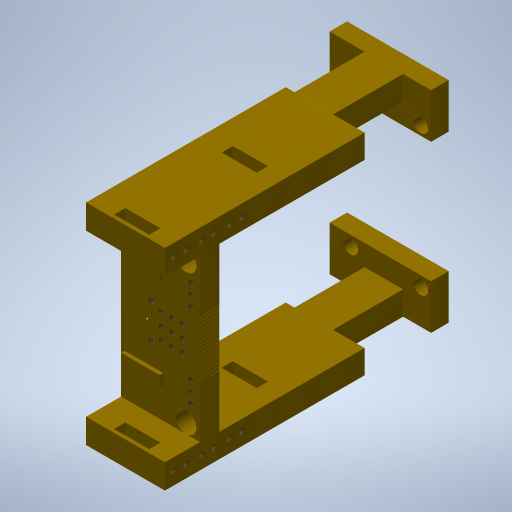
# Autodesk Inventor part: sample_holder_test
Saved by Autodesk Inventor 2024 (Build 280153000, 153)
## iProperties
Created: 2017-12-08
Part Number: sample_holder_test
Material: Generic
Document SubType Name: Modeling
Designer: awallucks
Density: 1 g/cm^3
Appearance: Default
Author: awallucks
Autodesk Inventor part; units mm, degrees
ref_plane "YZ Plane" through (0, 0, 0) normal (1, 0, 0) x (0, 1, 0)
ref_plane "XZ Plane" through (0, 0, 0) normal (0, 1, 0) x (-1, 0, 0)
ref_plane "XY Plane" through (0, 0, 0) normal (0, 0, 1) x (1, 0, 0)
sketch "Sketch1" plane through (0, 0, 0) normal (0, 1, 0) x (-1, 0, 0)
  line L0 (15, 30) -> (-15, 30)
  line L1 (-15, 30) -> (-15, -30)
  line L2 (-15, -30) -> (15, -30)
  line L3 (15, -30) -> (15, 30)
  point P0 (0, 0)
  dimension "d0" = 15
  dimension "d1" = 30
  dimension "d2" = 60
  dimension "d3" = 30
  constraints: 8 end point, 2 parallel, 1 horizontal, 1 perpendicular
  measures "d0" distance from line of L3 point (0, 0)
  measures "d1" distance between parallel lines of L1 L3
  measures "d2" distance between parallel lines of L2 L0
  measures "d3" distance from line of L0 point (0, 0)
extrude "Extrusion1" add sketch "Sketch1" along normal blind 72
sketch "Sketch2" plane through (0, 72, 0) normal (0, 1, 0) x (1, 0, 0)
  line L0 (15, 17.25) -> (15, -17.25)
  line L1 (-15, 30) -> (-15, -30) projected
  line L2 (15, 17.25) -> (-15, 17.25)
  line L3 (-15, 17.25) -> (-15, -17.25)
  line L4 (-15, -17.25) -> (15, -17.25)
  line L5 (15, -17.25) -> (15, 17.25)
  point P0 (0, 0)
  constraints: 10 end point, 2 parallel, 1 horizontal, 1 perpendicular, 1 point on line
extrude "Extrusion2" cut sketch "Sketch2" against normal blind 66.5
sketch "Sketch3" plane through (0, 72, 0) normal (0, 1, 0) x (1, 0, 0)
  circle A0 centre (11, -20) radius 2.15
  point P0 (0, 0)
  dimension "d15" = 20
  dimension "d16" = 11
  dimension "d17" = 4.3
  constraints: 1 centre point
  measures "d15" vertical distance of A0.centre point (0, 0)
  measures "d16" horizontal distance of A0.centre point (0, 0)
  measures "d17" diameter of A0
sketch "Sketch4" plane through (0, 72, 0) normal (0, 1, 0) x (1, 0, 0)
  point P0 (0, 0)
extrude "Extrusion3" cut sketch "Sketch3" against normal blind 50
pattern_linear "Rectangular Pattern1" count 2 spacing 20 along (-1, 0, 0) count 2 spacing 40 along (0, 0, -1) of "Extrusion3"
sketch "Sketch7" plane through (0, 5.5, 0) normal (0, 1, 0) x (1, 0, 0)
  line L0 (15, 17.25) -> (15, -17.25) projected
  line L1 (-15, -30) -> (15, -30) projected
  point P0 (0, 0)
  point P1 (1.2, -5)
  point P2 (1.2, 5)
  dimension "d47" = 13.8
  dimension "d51" = 10
  dimension "d85" = 5
  constraints: 1 vertical, 1 other
  measures "d47" distance from line of L0 point (1.2, -5)
  measures "d51" distance of point (1.2, -5) point (1.2, 5)
  measures "d85" vertical distance of point (0, 0) point (1.2, -5)
hole "Hole2" at (1.2, 5.5, 5) at (1.2, 5.5, -5) direction (0, -1, 0) diameter 1.567 depth 6.3 thread size "M2x0.4" class "6H" standard "ISO Metric profile"
sketch "Sketch10" plane through (15, 0, 30) normal (1, 0, 0) x (0, 0, -1)
  line L0 (0, 72) -> (12.75, 72)
  line L1 (12.75, 72) -> (12.75, 5.5)
  line L2 (12.75, 5.5) -> (0, 5.5)
  line L3 (0, 5.5) -> (0, 72)
  line L4 (60, 0) -> (60, 72) projected
  line L5 (47.25, 72) -> (60, 72)
  line L6 (60, 72) -> (60, 5.5)
  line L7 (60, 5.5) -> (47.25, 5.5)
  line L8 (47.25, 5.5) -> (47.25, 72)
  point P0 (30, 0)
  constraints: 16 end point, 4 parallel, 2 horizontal, 2 perpendicular, 2 point on line
extrude "Extrusion6" cut sketch "Sketch10" against normal blind 1
sketch "Sketch12" plane through (0, 0, 0) normal (0, -1, 0) x (1, 0, 0)
  line L0 (15, 6) -> (15, -6) projected
  line L1 (15, 30) -> (15, -30) projected
  point P0 (0, 0)
  point P1 (15, 0)
  point P2 (15, -1)
  point P3 (15, -2)
  point P4 (15, -3)
  point P5 (15, -4)
  point P6 (15, -5)
  point P7 (15, 0)
  point P8 (15, 1)
  point P9 (15, 2)
  point P10 (15, 3)
  point P11 (15, 4)
  point P12 (15, 5)
  point P13 (15, 0)
  point P14 (15, -7)
  point P15 (15, -8)
  point P16 (15, 7)
  point P17 (15, 8)
  dimension "d292" = 1
  dimension "d293" = 1
  dimension "d294" = 1
  dimension "d295" = 1
  dimension "d296" = 1
  constraints: 3 coincident, 15 other
  measures "d292" distance of point (15, 5) point (15, 6)
  measures "d293" distance of point (15, 7) point (15, 6)
  measures "d294" distance of point (15, -7) point (15, -6)
  measures "d295" distance of point (15, -8) point (15, -7)
  measures "d296" distance of point (15, 8) point (15, 7)
hole "Hole4" at (15, 0, 0) at (15, 0, -1) at (15, 0, -2) at (15, 0, -3) at (15, 0, 1) at (15, 0, 2) at (15, 0, 3) at (15, 0, -4) at (15, 0, -5) at (15, 0, 5) at (15, 0, 4) at (15, 0, 6) at (15, 0, -6) at (15, 0, -7) at (15, 0, -8) at (15, 0, 7) at (15, 0, 8) direction (0, 1, 0) diameter 0.2 end through all
sketch "Sketch14" plane through (15, 0, -30) normal (0, 0, -1) x (-1, 0, 0)
  line L0 (1, 67) -> (9, 67)
  line L1 (9, 67) -> (9, 47)
  line L2 (9, 47) -> (1, 47)
  line L3 (1, 47) -> (1, 67)
  line L4 (1, 67) -> (9, 47) construction
  line L5 (9, 67) -> (1, 47) construction
  line L6 (1, 72) -> (30, 72) projected
  line L7 (28, 47) -> (20, 47)
  line L8 (20, 47) -> (20, 67)
  line L9 (20, 67) -> (28, 67)
  line L10 (28, 67) -> (28, 47)
  line L11 (28, 47) -> (20, 67) construction
  line L12 (20, 47) -> (28, 67) construction
  line L13 (1, 72) -> (1, 5.5) projected
  line L14 (30, 0) -> (30, 72) projected
  point P0 (15, 0)
  point P1 (5, 57)
  point P2 (5, 67)
  point P3 (24, 57)
  point P4 (24, 47)
  dimension "d113" = 5
  dimension "d114" = 20
  dimension "d115" = 0
  dimension "d116" = 5
  dimension "d117" = 20
  dimension "d118" = 8
  dimension "d119" = 8
  dimension "d120" = 2
  constraints: 24 end point, 6 midpoint, 4 parallel, 2 horizontal, 2 perpendicular
  measures "d113" distance from line of point (5, 67) L6
  measures "d114" distance between parallel lines of L2 L0
  measures "d115" distance between parallel lines of L13 L3
  measures "d116" distance between parallel lines of L6 L9
  measures "d117" distance from line of point (24, 47) L9
  measures "d118" distance between parallel lines of L3 L1
  measures "d119" distance between parallel lines of L10 L8
  measures "d120" distance between parallel lines of L14 L10
extrude "Extrusion7" cut sketch "Sketch14" against normal blind 60
sketch "Sketch15" plane through (6, 47, 17.25) normal (0, 1, 0) x (1, 0, 0)
  line L0 (8, 0) -> (8, -12.75) projected
  line L1 (0, 0) -> (8, 0)
  line L2 (8, 0) -> (8, -6)
  line L3 (8, -6) -> (0, -6)
  line L4 (0, -6) -> (0, 0)
  line L5 (0, 0) -> (8, -6) construction
  line L6 (8, 0) -> (0, -6) construction
  line L7 (0, 0) -> (0, -12.75) projected
  line L8 (0, 0) -> (8, 0) projected
  line L9 (8, 40.5) -> (0, 40.5)
  line L10 (0, 40.5) -> (0, 34.5)
  line L11 (0, 34.5) -> (8, 34.5)
  line L12 (8, 34.5) -> (8, 40.5)
  line L13 (8, 40.5) -> (0, 34.5) construction
  line L14 (0, 40.5) -> (8, 34.5) construction
  line L15 (8, 34.5) -> (0, 34.5) projected
  line L16 (-19, 0) -> (-11, 0) projected
  line L17 (-19, -5.5) -> (-11, -5.5)
  line L18 (-11, -5.5) -> (-11, 0)
  line L19 (-11, 0) -> (-19, 0)
  line L20 (-19, 0) -> (-19, -5.5)
  circle A0 centre (-15, -2.75) radius 2.15 projected
  line L21 (-19, -5.5) -> (-11, 0) construction
  line L22 (-11, -5.5) -> (-19, 0) construction
  line L23 (-19, 34.25) -> (-11, 34.25)
  line L24 (-11, 34.25) -> (-11, 40.25)
  line L25 (-11, 40.25) -> (-19, 40.25)
  line L26 (-19, 40.25) -> (-19, 34.25)
  circle A1 centre (-15, 37.25) radius 2.15 projected
  line L27 (-19, 34.25) -> (-11, 40.25) construction
  line L28 (-11, 34.25) -> (-19, 40.25) construction
  point P0 (-6, 17.25)
  point P1 (4, -3)
  point P2 (4, 0)
  point P3 (4, 0)
  point P4 (4, 0)
  point P5 (4, -6)
  point P6 (4, 37.5)
  point P7 (4, 34.5)
  dimension "d121" = 0
  dimension "d122" = 0
  dimension "d123" = 6
  dimension "d126" = 6
  dimension "d127" = 0
  dimension "d128" = 8
  dimension "d129" = 6
  constraints: 48 end point, 13 midpoint, 8 parallel, 4 horizontal, 4 perpendicular, 1 point on line
  measures "d121" distance from line of L7 L1.start
  measures "d122" distance of point (4, 0) point (4, 0)
  measures "d123" distance of point (4, 0) point (4, -6)
  measures "d126" distance between parallel lines of L11 L9
  measures "d127" distance from line of L15 point (4, 34.5)
  measures "d128" distance of L25.end L24.end
  measures "d129" distance of L23.end L24.end
extrude "Extrusion8" cut sketch "Sketch15" against normal up to surface (41.5 mm away) contours L0 L3 L4 L1 | L12 L11 L10 L9 | L16 L18 L17 L20 | A0 | L26 L25 L24 L23 | A1
sketch "Sketch16" plane through (0, 5.5, 0) normal (0, 1, 0) x (1, 0, 0)
  circle A0 centre (11, 20) radius 2.15 projected
  circle A1 centre (11, 20) radius 3
  circle A2 centre (11, -20) radius 2.15 projected
  circle A3 centre (11, -20) radius 3
  point P0 (0, 0)
  dimension "d134" = 6
  dimension "d137" = 6
  constraints: 2 centre point, 2 coincident
  measures "d134" diameter of A1
  measures "d137" diameter of A3
extrude "Extrusion9" cut sketch "Sketch16" against normal through all contours A0 | A1 | A2 | A3
sketch "Sketch18" plane through (0, 0, 0) normal (0, -1, 0) x (1, 0, 0)
  line L0 (-15, 17.25) -> (-15, 30) projected
  line L1 (14, 23) -> (-15, 23)
  line L2 (-15, 23) -> (-15, 30)
  line L3 (-15, 30) -> (14, 30)
  line L4 (14, 30) -> (14, 23)
  line L5 (14, 23) -> (-15, 30) construction
  line L6 (-15, 23) -> (14, 30) construction
  line L7 (15, -30) -> (-15, -30) projected
  line L8 (14, -23) -> (-15, -23)
  line L9 (-15, -23) -> (-15, -30)
  line L10 (-15, -30) -> (14, -30)
  line L11 (14, -30) -> (14, -23)
  line L12 (14, -23) -> (-15, -30) construction
  line L13 (-15, -23) -> (14, -30) construction
  point P0 (0, 0)
  point P1 (-0.5, 26.5)
  point P2 (-0.5, -26.5)
  point P3 (-15, -26.5)
  point P4 (14, -26.5)
  point P5 (14, -30)
  dimension "d141" = 7
  dimension "d142" = 29
  dimension "d144" = 29
  dimension "d210" = 7
  constraints: 24 end point, 6 midpoint, 4 parallel, 2 horizontal, 2 perpendicular
  measures "d141" distance of L1.start L3.end
  measures "d142" distance of L1.end L1.start
  measures "d144" distance of point (-15, -26.5) point (14, -26.5)
  measures "d210" distance from line of L10.end L8
extrude "Extrusion10" add sketch "Sketch18" along normal blind 10
sketch "Sketch24" plane through (-15, 5.5, -17.25) normal (-1, 0, 0) x (0, 0, 1)
  line L0 (47.25, 61.5) -> (37.25, 61.5) projected
  line L1 (-12.75, -15.5) -> (-5.75, -15.5) projected
  line L2 (47.25, 61.5) -> (-12.75, 61.5)
  line L3 (-12.75, 61.5) -> (-12.75, -15.5)
  line L4 (-12.75, -15.5) -> (47.25, -15.5)
  line L5 (47.25, -15.5) -> (47.25, 61.5)
  line L6 (-12.75, -15.5) -> (-12.75, 66.5) projected
  point P0 (17.25, -5.5)
  point P1 (-5.75, -15.5)
  dimension "d214" = 0
  dimension "d215" = 0
  constraints: 8 end point, 2 parallel, 2 point on line, 1 horizontal, 1 perpendicular
  measures "d214" distance from line of L6 L2.end
  measures "d215" distance of L0.start L2.start
extrude "Extrusion13" cut sketch "Sketch24" against normal blind 7.5
sketch "Sketch26" plane through (-5, 5.5, -17.25) normal (-1, 0, 0) x (0, 0, 1)
  line L0 (0, 61.5) -> (-12.75, 61.5) projected
  line L1 (-6, 41.5) -> (-6, 0) projected
  line L2 (0, 61.5) -> (-6, 61.5)
  line L3 (-6, 61.5) -> (-6, 0)
  line L4 (-6, 0) -> (0, 0)
  line L5 (0, 0) -> (0, 61.5)
  line L6 (34.2811, 61.5) -> (40.5, 61.5)
  line L7 (40.5, 61.5) -> (40.5, 0)
  line L8 (40.5, 0) -> (34.2811, 0)
  line L9 (34.2811, 0) -> (34.2811, 61.5)
  point P0 (17.25, -5.5)
  point P1 (-6, 39.5)
  point P2 (-6, 61.5)
  point P3 (-6, 39.5)
  constraints: 16 end point, 4 parallel, 2 horizontal, 2 perpendicular
extrude "Extrusion14" cut sketch "Sketch26" against normal through all
sketch "Sketch27" plane through (14, 0, 30) normal (1, 0, 0) x (0, 0, -1)
  line L0 (0, 0) -> (24.9, 0) projected
  line L1 (0, 0) -> (7, 0)
  line L2 (7, 0) -> (7, -10)
  line L3 (7, -10) -> (0, -10)
  line L4 (0, -10) -> (0, 0)
  line L5 (35.1, 0) -> (60, 0) projected
  line L6 (60, 0) -> (53, 0)
  line L7 (53, 0) -> (53, -10)
  line L8 (53, -10) -> (60, -10)
  line L9 (60, -10) -> (60, 0)
  point P0 (30, 0)
  constraints: 16 end point, 4 parallel, 2 horizontal, 2 perpendicular
extrude "Extrusion15" add sketch "Sketch27" along normal blind 1
sketch "Sketch28" plane through (-15, 72, 30) normal (0, 0, 1) x (1, 0, 0)
  line L0 (24.5, -77.8) -> (14.5, -77.8)
  line L1 (14.5, -77.8) -> (14.5, -81)
  line L2 (14.5, -81) -> (24.5, -81)
  line L3 (24.5, -81) -> (24.5, -77.8)
  line L4 (30, -82) -> (30, -66.5) projected
  line L5 (7.5, -82) -> (30, -82) projected
  line L6 (14.5, -47.1) -> (24.5, -47.1)
  line L7 (24.5, -47.1) -> (24.5, -50.3)
  line L8 (24.5, -50.3) -> (14.5, -50.3)
  line L9 (14.5, -50.3) -> (14.5, -47.1)
  point P0 (24.5, -79.4)
  point P1 (14.5, -79.4)
  dimension "d222" = 3.2
  dimension "d223" = 5.5
  dimension "d224" = 10
  dimension "d225" = 1
  dimension "d242" = 10
  dimension "d243" = 3.2
  dimension "d244" = 27.5
  constraints: 16 end point, 4 parallel, 2 horizontal, 2 midpoint, 2 perpendicular
  measures "d222" distance of L2.end L0.start
  measures "d223" distance from line of L4 point (24.5, -79.4)
  measures "d224" distance of point (24.5, -79.4) point (14.5, -79.4)
  measures "d225" distance between parallel lines of L5 L2
  measures "d242" distance of L7.end L8.end
  measures "d243" distance of L6.end L7.end
  measures "d244" distance between parallel lines of L0 L8
extrude "Extrusion16" cut sketch "Sketch28" against normal through all
sketch "Sketch30" plane through (-7.5, 5.5, -23) normal (0, 0, 1) x (1, 0, 0)
  line L0 (0, 41.5) -> (0, 0) projected
  line L1 (2.5, 41.5) -> (2.5, 0) projected
  line L2 (0, 41.5) -> (2.5, 41.5)
  line L3 (2.5, 41.5) -> (2.5, 0)
  line L4 (2.5, 0) -> (0, 0)
  line L5 (0, 0) -> (0, 41.5)
  point P0 (7.5, -5.5)
  constraints: 8 end point, 2 parallel, 1 horizontal, 1 perpendicular
extrude "Extrusion17" cut sketch "Sketch30" against normal blind 0.25
sketch "Sketch32" plane through (-7.5, 5.5, 22.75) normal (0, 0, -1) x (-1, 0, 0)
  line L0 (-2.5, 41.5) -> (-2.5, 0) projected
  line L1 (0, 0) -> (-2.5, 0) projected
  line L2 (-2.5, 41.5) -> (0, 41.5)
  line L3 (0, 41.5) -> (0, 0)
  line L4 (0, 0) -> (-2.5, 0)
  line L5 (-2.5, 0) -> (-2.5, 41.5)
  point P0 (-7.5, -5.5)
  constraints: 8 end point, 2 parallel, 1 horizontal, 1 perpendicular
extrude "Extrusion19" cut sketch "Sketch32" against normal blind 0.5
sketch "Sketch33" plane through (14, 0, 30) normal (1, 0, 0) x (0, 0, -1)
  line L0 (0, 5.5) -> (0, 47) projected
  line L1 (6.75, 5.5) -> (53.25, 5.5) projected
  line L2 (0, 47) -> (6.75, 47)
  line L3 (6.75, 47) -> (6.75, 5.5)
  line L4 (6.75, 5.5) -> (0, 5.5)
  line L5 (0, 5.5) -> (0, 47)
  line L6 (60, 47) -> (60, 5.5) projected
  line L7 (53.25, 47) -> (60, 47)
  line L8 (60, 47) -> (60, 5.5)
  line L9 (60, 5.5) -> (53.25, 5.5)
  line L10 (53.25, 5.5) -> (53.25, 47)
  point P0 (30, 0)
  constraints: 16 end point, 4 parallel, 2 horizontal, 2 perpendicular
extrude "Extrusion20" add sketch "Sketch33" along normal blind 1
sketch "Sketch29" plane through (15, 0, 5.1) normal (1, 0, 0) x (0, 0, -1)
  line L0 (-24.9, -10) -> (-24.9, 5.5) projected
  line L1 (-24.9, -10) -> (-17.9, -10) projected
  line L2 (35.1, -10) -> (35.1, 5.5) projected
  line L3 (28.1, -10) -> (35.1, -10) projected
  point P0 (5.1, 0)
  point P1 (-21.4, -7.5)
  point P2 (-21.4, -4)
  point P3 (-21.4, -10)
  point P4 (31.6, -4)
  point P5 (31.6, -7.5)
  point P6 (-21.4, 0.5)
  point P7 (-21.4, 4)
  point P8 (31.6, 4)
  point P9 (31.6, 0.5)
  point P10 (-21.4, 8.5)
  point P11 (-21.4, 12)
  point P12 (31.6, 12)
  point P13 (31.6, 8.5)
  dimension "d235" = 3.5
  dimension "d236" = 3.5
  dimension "d237" = 2.5
  dimension "d238" = 3.5
  dimension "d239" = 3.5
  dimension "d240" = 3.5
  dimension "d241" = 2.5
  dimension "d253" = 3.5
  dimension "d254" = 4.5
  dimension "d255" = 3.5
  dimension "d256" = 4.5
  dimension "d257" = 3.5
  dimension "d258" = 3.5
  dimension "d259" = 4.5
  dimension "d260" = 4.5
  constraints: 1 midpoint
  measures "d235" distance from line of L0 point (-21.4, -4)
  measures "d236" distance of point (-21.4, -4) point (-21.4, -7.5)
  measures "d237" distance of point (-21.4, -10) point (-21.4, -7.5)
  measures "d238" distance from line of L2 point (31.6, -4)
  measures "d239" distance from line of L2 point (31.6, -7.5)
  measures "d240" distance of point (31.6, -4) point (31.6, -7.5)
  measures "d241" distance from line of L3 point (31.6, -7.5)
  measures "d253" distance of point (-21.4, 4) point (-21.4, 0.5)
  measures "d254" distance of point (-21.4, -4) point (-21.4, 0.5)
  measures "d255" distance of point (31.6, 4) point (31.6, 0.5)
  measures "d256" distance of point (31.6, -4) point (31.6, 0.5)
  measures "d257" distance of point (-21.4, 12) point (-21.4, 8.5)
  measures "d258" distance of point (31.6, 12) point (31.6, 8.5)
  measures "d259" distance of point (31.6, 8.5) point (31.6, 4)
  measures "d260" distance of point (-21.4, 4) point (-21.4, 8.5)
hole "Hole8" at (15, -7.5, 26.5) at (15, -4, 26.5) at (15, -4, -26.5) at (15, -7.5, -26.5) at (15, 0.5, 26.5) at (15, 4, 26.5) at (15, 0.5, -26.5) at (15, 4, -26.5) at (15, 8.5, 26.5) at (15, 12, 26.5) at (15, 8.5, -26.5) at (15, 12, -26.5) direction (-1, 0, 0) diameter 1.567 depth 5 tip angle 118 thread size "M2x0.4" class "6H" standard "ISO Metric profile"
sketch "Sketch34" plane through (0, 5.5, 0) normal (0, 1, 0) x (1, 0, 0)
  line L0 (-7.5, -23) -> (-7.5, 23) projected
  line L1 (-7.5, 7) -> (-6, 7)
  line L2 (-6, 7) -> (-6, 15)
  line L3 (-6, 15) -> (-7.5, 15)
  line L4 (-7.5, 15) -> (-7.5, 7)
  line L5 (-6, -7) -> (-7.5, -7)
  line L6 (-7.5, -7) -> (-7.5, -15)
  line L7 (-7.5, -15) -> (-6, -15)
  line L8 (-6, -15) -> (-6, -7)
  line L9 (-7.5, -23.25) -> (-7.5, 23.25) projected
  point P0 (0, 0)
  point P1 (-7.5, -7)
  point P2 (-7.5, -15)
  point P3 (-7.5, 15)
  point P4 (-7.5, 0)
  point P5 (-7.5, 0)
  dimension "d263" = 1.5
  dimension "d264" = 7
  dimension "d265" = 7
  dimension "d266" = 8
  dimension "d267" = 8
  constraints: 16 end point, 4 parallel, 3 point on line, 2 horizontal, 2 perpendicular, 1 midpoint, 2 other
  measures "d263" distance of L1.start L1.end
  measures "d264" distance of L5.end point (-7.5, 0)
  measures "d265" distance of L1.start point (-7.5, 0)
  measures "d266" distance of L2.end L1.end
  measures "d267" distance of L5.start L7.end
extrude "Extrusion21" add sketch "Sketch34" along normal blind 15
sketch "Sketch35" plane through (-7.5, 5.5, -17.25) normal (-1, 0, 0) x (0, 0, 1)
  line L0 (4.65, 13) -> (7.85, 13)
  line L1 (7.85, 13) -> (7.85, 2)
  line L2 (7.85, 2) -> (4.65, 2)
  line L3 (4.65, 2) -> (4.65, 13)
  line L4 (26.65, 13) -> (29.85, 13)
  line L5 (29.85, 13) -> (29.85, 2)
  line L6 (29.85, 2) -> (26.65, 2)
  line L7 (26.65, 2) -> (26.65, 13)
  line L8 (2.25, 0) -> (2.25, 15) projected
  line L9 (24.25, 0) -> (24.25, 15) projected
  line L10 (2.25, 15) -> (10.25, 15) projected
  line L11 (2.25, 0) -> (10.25, 0) projected
  line L12 (24.25, 15) -> (32.25, 15) projected
  line L13 (24.25, 0) -> (32.25, 0) projected
  point P0 (17.25, -5.5)
  point P1 (6.25, 2)
  point P2 (28.25, 13)
  point P3 (28.25, 2)
  dimension "d268" = 3.2
  dimension "d270" = 3.2
  dimension "d272" = 4
  dimension "d273" = 4
  dimension "d276" = 2
  dimension "d277" = 2
  dimension "d278" = 2
  dimension "d279" = 2
  constraints: 16 end point, 4 parallel, 3 midpoint, 2 horizontal, 2 perpendicular
  measures "d268" distance of L1.end L2.end
  measures "d270" distance of L5.end L6.end
  measures "d272" distance from line of L8 point (6.25, 2)
  measures "d273" distance from line of L9 point (28.25, 13)
  measures "d276" distance between parallel lines of L10 L0
  measures "d277" distance between parallel lines of L11 L2
  measures "d278" distance between parallel lines of L12 L4
  measures "d279" distance from line of L13 point (28.25, 2)
extrude "Extrusion22" cut sketch "Sketch35" against normal through all
sketch "Sketch36" plane through (0, 0, 0) normal (0, -1, 0) x (1, 0, 0)
  line L0 (4.5, 14.7857) -> (-6.5, 14.7857)
  line L1 (-6.5, 14.7857) -> (-6.5, 11.7857)
  line L2 (-6.5, 11.7857) -> (4.5, 11.7857)
  line L3 (4.5, 11.7857) -> (4.5, 14.7857)
  line L4 (4.5, -11.1857) -> (-6.5, -11.1857)
  line L5 (-6.5, -11.1857) -> (-6.5, -14.1857)
  line L6 (-6.5, -14.1857) -> (4.5, -14.1857)
  line L7 (4.5, -14.1857) -> (4.5, -11.1857)
  line L8 (-7.5, 23) -> (-7.5, -23) projected
  point P0 (0, 0)
  point P1 (-6.5, 13.2857)
  point P2 (-6.5, -12.6857)
  dimension "d280" = 3
  dimension "d281" = 11
  dimension "d282" = 1
  dimension "d283" = 1
  dimension "d284" = 3
  dimension "d285" = 11
  constraints: 16 end point, 4 parallel, 2 horizontal, 2 midpoint, 2 perpendicular, 2 point on line
  measures "d280" distance of L2.end L0.start
  measures "d281" distance of L0.end L0.start
  measures "d282" distance from line of L8 point (-6.5, 13.286)
  measures "d283" distance from line of L8 point (-6.5, -12.686)
  measures "d284" distance of L4.start L6.end
  measures "d285" distance of L4.end L4.start
extrude "Extrusion23" add sketch "Sketch36" along normal blind 1
sketch "Sketch38" plane through (0, 0, 0) normal (0, -1, 0) x (1, 0, 0)
  point P0 (0, 0)
sketch "Sketch39" plane through (0, 0, 0) normal (0, -1, 0) x (1, 0, 0)
  line L0 (15, 0.1) -> (15, 0.9) projected
  line L1 (15, -0.9) -> (15, -0.1) projected
  line L2 (15, -1.9) -> (15, -1.1) projected
  line L3 (15, -2.9) -> (15, -2.1) projected
  line L4 (15, -3.9) -> (15, -3.1) projected
  line L5 (15, -4.9) -> (15, -4.1) projected
  line L6 (15, -5.9) -> (15, -5.1) projected
  line L7 (15, -6.9) -> (15, -6.1) projected
  line L8 (15, -7.9) -> (15, -7.1) projected
  line L9 (15, 1.1) -> (15, 1.9) projected
  line L10 (15, 2.1) -> (15, 2.9) projected
  line L11 (15, 3.1) -> (15, 3.9) projected
  line L12 (15, 4.9) -> (15, 4.1) projected
  line L13 (15, 5.9) -> (15, 5.1) projected
  line L14 (15, 6.9) -> (15, 6.1) projected
  line L15 (15, 7.1) -> (15, 7.9) projected
  point P0 (0, 0)
  point P1 (15, 0.5)
  point P2 (15, -0.5)
  point P3 (15, -1.5)
  point P4 (15, -2.5)
  point P5 (15, -3.5)
  point P6 (15, -4.5)
  point P7 (15, -5.5)
  point P8 (15, -6.5)
  point P9 (15, -7.5)
  point P10 (15, 1.5)
  point P11 (15, 2.5)
  point P12 (15, 3.5)
  point P13 (15, 4.5)
  point P14 (15, 5.5)
  point P15 (15, 6.5)
  point P16 (15, 7.5)
  constraints: 16 midpoint
hole "Hole9" at (15, 0, 7.5) at (15, 0, 6.5) at (15, 0, 5.5) at (15, 0, 4.5) at (15, 0, 3.5) at (15, 0, 2.5) at (15, 0, 1.5) at (15, 0, 0.5) at (15, 0, -0.5) at (15, 0, -1.5) at (15, 0, -2.5) at (15, 0, -3.5) at (15, 0, -4.5) at (15, 0, -5.5) at (15, 0, -6.5) at (15, 0, -7.5) direction (0, 1, 0) diameter 0.1 end through all
sketch "Sketch40" plane through (0, 0, 0) normal (0, -1, 0) x (1, 0, 0)
  line L0 (15, 23) -> (15, 8.1) projected
  line L1 (15, -8.1) -> (15, -23) projected
  line L2 (15, -3.1) -> (15, -3.45) projected
  line L3 (-7.5, -30) -> (15, -30) projected
  line L4 (-7.5, 30) -> (15, 30) projected
  point P0 (0, 0)
  point P1 (12.5, 15)
  point P2 (12.5, 12)
  point P3 (12.5, 9)
  point P4 (12.5, -9)
  point P5 (12.5, -12)
  point P6 (12.5, -15)
  point P7 (10, 3.5)
  point P8 (15, -3.275)
  point P9 (10, 0)
  point P10 (10, -3.5)
  point P11 (7, 3.5)
  point P12 (7, 0)
  point P13 (7, -3.5)
  point P14 (4, 3.5)
  point P15 (4, 0)
  point P16 (4, -3.5)
  dimension "d304" = 3
  dimension "d305" = 3
  dimension "d306" = 2.5
  dimension "d307" = 2.5
  dimension "d308" = 2.5
  dimension "d309" = 2.5
  dimension "d310" = 2.5
  dimension "d311" = 2.5
  dimension "d312" = 3
  dimension "d313" = 3
  dimension "d320" = 5
  dimension "d323" = 3.5
  dimension "d328" = 26.5
  dimension "d338" = 3
  dimension "d343" = 15
  dimension "d344" = 15
  constraints: 1 horizontal, 1 midpoint, 1 vertical, 8 other
  measures "d304" distance of point (12.5, 12) point (12.5, 9)
  measures "d305" distance of point (12.5, 15) point (12.5, 12)
  measures "d306" distance from line of L0 point (12.5, 12)
  measures "d307" distance from line of L0 point (12.5, 9)
  measures "d308" distance from line of L0 point (12.5, 15)
  measures "d309" distance from line of L1 point (12.5, -9)
  measures "d310" distance from line of L1 point (12.5, -12)
  measures "d311" distance from line of L1 point (12.5, -15)
  measures "d312" distance of point (12.5, -12) point (12.5, -15)
  measures "d313" distance of point (12.5, -9) point (12.5, -12)
  measures "d320" horizontal distance of point (15, -3.275) point (10, 3.5)
  measures "d323" distance of point (10, 3.5) point (10, 0)
  measures "d328" distance from line of L3 point (10, -3.5)
  measures "d338" distance of point (10, 3.5) point (7, 3.5)
  measures "d343" distance from line of L4 point (12.5, 15)
  measures "d344" distance from line of L3 point (12.5, -15)
hole "Hole10" at (12.5, 0, 15) at (12.5, 0, 12) at (12.5, 0, 9) at (12.5, 0, -9) at (12.5, 0, -12) at (12.5, 0, -15) at (10, 0, 3.5) at (10, 0, 0) at (10, 0, -3.5) at (7, 0, 3.5) at (7, 0, 0) at (7, 0, -3.5) at (4, 0, 3.5) at (4, 0, 0) at (4, 0, -3.5) direction (0, 1, 0) diameter 1.567 end through all thread size "M2x0.4" class "6H" standard "ISO Metric profile"
body "Solid1"
